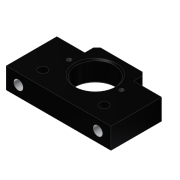
# Autodesk Inventor part: Lagerbock_Loslager
Saved by Autodesk Inventor 2016 (Build 200138000, 138)
## iProperties
Created: 2015-07-24
Part Number: Lagerbock_Loslager
Material: Aluminum 6061
Document SubType Name: Modeling
Density: 2.71 g/cm^3
Appearance: Smooth - Black
Autodesk Inventor part; units mm, degrees
ref_plane "YZ Plane" through (0, 0, 0) normal (1, 0, 0) x (0, 1, 0)
ref_plane "XZ Plane" through (0, 0, 0) normal (0, 1, 0) x (-1, 0, 0)
ref_plane "XY Plane" through (0, 0, 0) normal (0, 0, 1) x (1, 0, 0)
sketch "Sketch1" plane through (0, 0, 0) normal (0, 0, 1) x (1, 0, 0)
  line L0 (-30, 0) -> (30, 0)
  line L1 (30, 0) -> (30, 29)
  line L2 (30, 29) -> (14, 29)
  line L3 (14, 29) -> (14, 36)
  line L4 (14, 36) -> (-14, 36)
  line L5 (-14, 36) -> (-14, 29)
  line L6 (-14, 29) -> (-30, 29)
  line L7 (-30, 29) -> (-30, 0)
  point P0 (0, 0)
  point P1 (0, 0)
  dimension "d0" = 60
  dimension "d1" = 36
  dimension "d2" = 7
  dimension "d3" = 28
  constraints: 16 end point, 6 perpendicular, 2 point on line, 1 coincident, 1 collinear, 1 horizontal, 1 midpoint
  measures "d0" distance between parallel lines of L1 L7
  measures "d1" distance between parallel lines of L0 L4
  measures "d2" distance between parallel lines of L6 L4
  measures "d3" distance of L3.end L4.end
extrude "Extrusion1" add sketch "Sketch1" along normal mid plane 12
sketch "Sketch2" plane through (0, 0, 6) normal (0, 0, 1) x (1, 0, 0)
  line L0 (-30, 0) -> (30, 0) projected
  point P0 (0, 0)
  point P1 (0, 21)
  point P2 (0, 0)
  dimension "d6" = 21
  constraints: 1 midpoint, 1 vertical alignment
  measures "d6" distance from line of L0 point (0, 21)
hole "Hole1" at (0, 21, 6) direction (0, 0, -1) diameter 22 end through all
chamfer "Chamfer1" distance 0.8 angle 45 2 edges at (0, 32, 6) (0, 32, -6)
chamfer "Chamfer2" distance 2 angle 45 2 edges at (-14, 36, 0) (14, 36, 0)
sketch "Sketch3" plane through (-30, 29, 6) normal (0, 1, 0) x (1, 0, 0)
  line L0 (0, 12) -> (0, 0) projected
  line L1 (60, 12) -> (60, 0) projected
  point P0 (30, 6)
  point P1 (7, 6)
  point P2 (52.5, 6)
  dimension "d20" = 45.5
  dimension "d21" = 7
  dimension "d22" = 7.5
  constraints: 2 horizontal alignment
  measures "d20" distance of point (52.5, 6) point (7, 6)
  measures "d21" distance from line of L0 point (7, 6)
  measures "d22" distance from line of L1 point (52.5, 6)
hole "Hole2" at (-23, 29, 0) at (22.5, 29, 0) direction (0, -1, 0) diameter 5.5 end through all counterbore diameter 9 counterbore depth 6
sketch "Sketch4" plane through (0, 0, 6) normal (0, 0, 1) x (1, 0, 0)
  line L0 (-30, 0) -> (30, 0) projected
  line L1 (-30, 29) -> (-30, 0) projected
  point P0 (0, 0)
  point P1 (-17.5, 8.5)
  point P2 (17.5, 8.5)
  dimension "d30" = 35
  dimension "d31" = 8.5
  dimension "d32" = 12.5
  constraints: 1 horizontal alignment
  measures "d30" distance of point (-17.5, 8.5) point (17.5, 8.5)
  measures "d31" distance from line of L0 point (-17.5, 8.5)
  measures "d32" distance from line of L1 point (-17.5, 8.5)
hole "Hole3" at (-17.5, 8.5, 6) at (17.5, 8.5, 6) direction (0, 0, -1) diameter 5 end through all
sketch "Sketch5" plane through (0, 0, 6) normal (0, 0, 1) x (1, 0, 0)
  circle A0 centre (0, 21) radius 11 projected
  circle A1 centre (0, 21) radius 11 projected
  point P0 (0, 0)
  point P1 (-15, 21)
  point P2 (15, 21)
  dimension "d40" = 30
  dimension "d41" = 15
  constraints: 2 horizontal alignment
  measures "d40" distance of point (15, 21) point (-15, 21)
  measures "d41" distance of point (15, 21) A0.centre
hole "Hole4" at (-15, 21, 6) at (15, 21, 6) direction (0, 0, -1) diameter 2.459 depth 10 tip angle 118 thread size "M3x0.5" designation "M3" class "6H" standard "ISO Metric profile"
equation "\"d41\" = 0.5 * d40"
body "Solid1"
